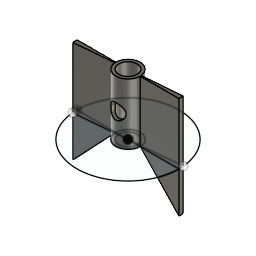
Agitator (Autodesk Fusion 360 design; units mm, degrees)
Autodesk Fusion 360 part; units mm, degrees
sketch "Sketch1" plane through (0, 0, 0) normal (0, 0, 1) x (1, 0, 0)
  circle A0 centre (0, 0) radius 33.5
  circle A1 centre (0, 0) radius 8
  circle A2 centre (0, 0) radius 6
  line L0 (0, 0) -> (33.5, 0)
  line L1 (0, 0) -> (33.3725, 2.9197)
  line L2 (0, 0) -> (-33.3725, -2.9197)
  line L3 (0, 0) -> (-33.5, 0)
  dimension "d1" = 67
  dimension "d2" = 16
  dimension "d3" = 12
  dimension "d4" = 175
  dimension "d31" = 360
  constraint coincident A0.centre A1.centre
  constraint coincident A0 L0.end
  constraint horizontal L0
  measures "d1" diameter of A0
  measures "d2" diameter of A1
  measures "d3" diameter of A2
  measures "d4" angle of L0 L1
extrude "Extrude1" add sketch "Sketch1" along normal blind 40 contours A1 A2 L0 L1 | A1 A2 L0 L2 | A1 A2 L1 L3 | A1 A2 L2 L3 | A2 L0 L1 | A2 L0 L2 | A2 L1 L3 | A2 L2 L3
shell "Shell1" thickness 2 removed faces 2 at (1.4678, 2.567, 40) at (1.4678, 2.567, 0)
sketch "Sketch2" plane through (0, 0, 0) normal (0, 1, 0) x (1, 0, 0)
  line L0 (8, 0) -> (8, -20) construction
  line L1 (8, -20) -> (0, -20) construction
  circle A0 centre (0, -20) radius 5
  line L2 (8, 0) -> (8, 27) construction
  line L3 (8, -40) -> (33.5, -40)
  line L4 (33.5, -40) -> (33.5, 27)
  line L5 (8, 0) -> (8, -40)
  line L6 (8, 0) -> (33.5, 27)
  line L7 (8, 0) -> (8, 27)
  line L8 (8, 27) -> (33.5, 27)
  dimension "d8" = 20
  dimension "d9" = 10
  dimension "d12" = 27
  dimension "d13" = 25.5
  constraint vertical L0
  constraint perpendicular L0 L1
  constraint coincident L1.end A0.centre
  constraint parallel L0 L2
  constraint horizontal L3
  constraint vertical L4
  constraint vertical L5
  measures "d8" distance of L0.start L0.end
  measures "d9" diameter of A0
  measures "d12" distance of L0.start L2.end
  measures "d13" distance of L3.start L3.end
extrude "Extrude2" cut sketch "Sketch2" along normal through all and the other way through all contours A0
extrude "Extrude3" add sketch "Sketch1" along normal blind 40 and the other way blind 27 contours A0 A1 L0 L1
extrude "Extrude4" cut sketch "Sketch2" along normal blind 4 contours L6 L7 L8
extrude "Extrude5" cut 1 faces at (8, 0.2333, -18) along direction (-1, 0, 0) blind 2
extrude "Extrude6" add sketch "Sketch1" along normal blind 43 contours A0 A1 L0 L1
pattern_circular "C-Pattern1" count 2 over 360 about axis through (0, 0, 1.75) along (0, 0, 1) of 6 faces at (24.9941, 0.4023, 43) (25, 0, 5.3333) (33.4681, 1.4612, 19.6779) (24.915, 2.1798, 5.3783) (24.9336, 1.9369, -17.9297) (7.9996, 0.0776, 41)
extrude "Extrude7" cut sketch "Sketch1" along normal blind 43 and the other way blind -40 contours A0 A1 L0 L1
extrude "Extrude8" cut sketch "Sketch1" along normal blind 45 and the other way blind -40 contours A0 A1 L2 L3
